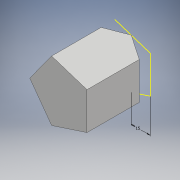
# Autodesk Inventor part: Призма
Saved by Autodesk Inventor 2018 (Build 220112000, 112)
## iProperties
Created: 2018-05-16
Part Number: Призма
Material: Типовые
Document SubType Name: Modeling
Designer: user
Density: 1 g/cm^3
Appearance: По умолчанию
Author: user
Autodesk Inventor part; units mm, degrees
ref_plane "YZ Plane" through (0, 0, 0) normal (1, 0, 0) x (0, 1, 0)
ref_plane "XZ Plane" through (0, 0, 0) normal (0, 1, 0) x (-1, 0, 0)
ref_plane "XY Plane" through (0, 0, 0) normal (0, 0, 1) x (1, 0, 0)
sketch "Эскиз3" plane through (0, 0, 0) normal (1, 0, 0) x (0, 1, 0)
  line L0 (50, 7.7254) -> (50, -20.2254) projected
  line L1 (50, -6.25) -> (41.9313, -20.2254)
  line L2 (50, -6.25) -> (23.7781, 25)
  line L3 (50, 25) -> (50, 7.7254) projected
  line L4 (0, -20.2254) -> (50, -20.2254) projected
  line L5 (0, 25) -> (50, 25) projected
  line L6 (23.7781, 25) -> (25, -20.2254)
  point P0 (0, 0)
  dimension "d4" = 140
  dimension "d5" = 150
  constraints: 6 end point, 2 midpoint, 2 point on line
  measures "d4" angle of L0 L2
  measures "d5" angle of L3 L1
extrude "Выдавливание2" [suppressed]
sketch "Эскиз4" plane through (0, 0, 0) normal (1, 0, 0) x (0, 1, 0)
  line L0 (50, -20.2254) -> (50, -6.25) projected
  line L1 (50, -6.25) -> (41.9313, -20.2254)
  line L2 (0, -20.2254) -> (50, -20.2254) projected
  line L3 (50, -6.25) -> (66.1374, -6.25) construction
  point P0 (0, 0)
  dimension "d8" = 120
  constraints: 4 end point, 1 equal length, 1 horizontal, 1 point on line
  measures "d8" angle of L1 L3
extrude "Выдавливание3" [suppressed]
sketch "Эскиз5" plane through (0, 0, 0) normal (0, 1, 0) x (-1, 0, 0)
  circle A0 centre (0, 0) radius 25
  line L0 (25, 0) -> (7.7254, -23.7764)
  line L1 (7.7254, -23.7764) -> (-20.2254, -14.6946)
  line L2 (-20.2254, -14.6946) -> (-20.2254, 14.6946)
  line L3 (-20.2254, 14.6946) -> (7.7254, 23.7764)
  line L4 (7.7254, 23.7764) -> (25, 0)
  dimension "d11" = 50
  constraints: 10 end point, 2 coincident, 1 horizontal alignment, 13 other
extrude "Выдавливание4" add sketch "Эскиз5" along normal blind 50 contours L0 L1 L2 L3 L4
sketch "Эскиз6" plane through (0, 50, 0) normal (0, 1, 0) x (1, 0, 0)
  line L0 (-7.7254, -23.7764) -> (20.2254, -14.6946) projected
  line L1 (5.2254, -19.5684) -> (5.2254, 19.5684)
  line L2 (20.2254, 14.6946) -> (-7.7254, 23.7764) projected
  line L3 (20.2254, -14.6946) -> (20.2254, 14.6946) projected
  point P0 (0, 0)
  dimension "d14" = 15
  constraints: 2 end point, 2 point on line, 1 vertical
  measures "d14" distance between parallel lines of L3 L1
sketch "Эскиз7" plane through (0, 0, 0) normal (0, 0, 1) x (1, 0, 0)
  line L0 (-7.7254, 50) -> (20.2254, 50) projected
  line L1 (20.2254, 50) -> (5.2254, 50)
  line L2 (5.2254, 50) -> (20.2254, 41.3397)
  line L3 (20.2254, 0) -> (20.2254, 50) projected
  line L4 (5.2254, 50) -> (22.5459, 50) construction
  line L5 (20.2254, 41.3397) -> (20.2254, 50)
  point P0 (0, 0)
  dimension "d15" = 15
  dimension "d16" = 30
  constraints: 8 end point, 2 point on line, 1 collinear, 1 equal length, 1 horizontal
  measures "d15" distance of L0.end L1.end
  measures "d16" angle of L2 L4
extrude "Выдавливание5" cut sketch "Эскиз7" along normal mid plane 50
sketch "Эскиз8" plane through (0, 0, 0) normal (0, 0, 1) x (1, 0, 0)
  line L0 (-25, 50) -> (-7.7254, 50) projected
  line L1 (-25, 50) -> (5.2254, 50)
  line L2 (5.2254, 50) -> (-25, 24.6379)
  line L3 (-25, 0) -> (-25, 50) projected
  line L4 (-25, 24.6379) -> (-25, 50)
  point P0 (0, 0)
  dimension "d19" = 40
  constraints: 6 end point, 1 collinear
  measures "d19" angle of L1 L2
extrude "Выдавливание6" cut sketch "Эскиз8" along normal mid plane 50
